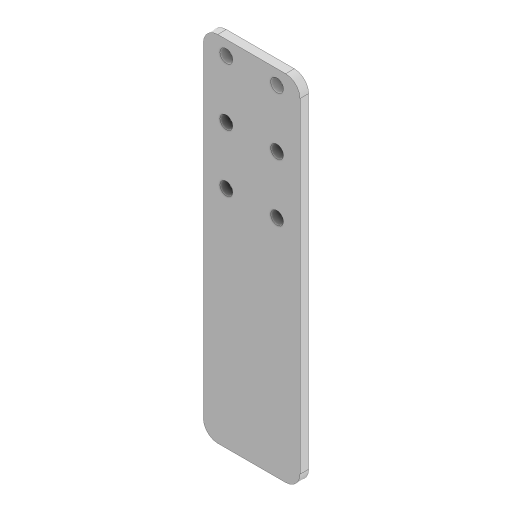
# Autodesk Inventor part: Lower Leaf
Saved by Autodesk Inventor 2024 (Build 280153000, 153)
## iProperties
Created: 2025-04-26
Part Number: Lower Leaf
Material: Generic
Document SubType Name: Modeling
Designer: Binara
Density: 1 g/cm^3
Appearance: Default
Author: Binara
Autodesk Inventor part; units mm, degrees
ref_plane "YZ Plane" through (0, 0, 0) normal (1, 0, 0) x (0, 1, 0)
ref_plane "XZ Plane" through (0, 0, 0) normal (0, 1, 0) x (-1, 0, 0)
ref_plane "XY Plane" through (0, 0, 0) normal (0, 0, 1) x (1, 0, 0)
sketch "Block1" plane through (0, 0, 0) normal (0, 0, 1) x (1, 0, 0)
  line L0 (22.2625, 0.2735) -> (22.2625, -13.7265)
  line L1 (56.7335, -13.7265) -> (22.2625, -13.7265)
  circle A0 centre (36.0618, -8.7265) radius 2.25
  circle A1 centre (53.7335, -8.7265) radius 2.25
  line L2 (61.7335, 0.2735) -> (61.7335, -8.7265)
  arc A2 (56.7335, -13.7265) -> (61.7335, -8.7265) centre (56.7335, -8.7265) ccw
  circle A3 centre (53.7335, 11.2735) radius 2.25
  line L3 (61.7335, 20.2735) -> (61.7335, 2.2735)
  circle A4 centre (36.0618, 11.2735) radius 2.25
  line L4 (61.7335, 0.2735) -> (22.2625, 0.2735)
  line L5 (22.2625, 2.2735) -> (61.7335, 2.2735)
  line L6 (22.2625, 20.2735) -> (22.2625, 2.2735)
  line L7 (61.7335, 31.2735) -> (61.7335, 22.2735)
  line L8 (61.7335, 20.2735) -> (22.2625, 20.2735)
  line L9 (22.2625, 22.2735) -> (61.7335, 22.2735)
  circle A5 centre (36.0618, 31.2735) radius 2.25
  line L10 (56.7335, 36.2735) -> (22.2625, 36.2735)
  line L11 (22.2625, 36.2735) -> (22.2625, 22.2735)
  circle A6 centre (53.7335, 31.2735) radius 2.25
  arc A7 (61.7335, 31.2735) -> (56.7335, 36.2735) centre (56.7335, 31.2735) ccw
  point P0 (44.3211, 11.7121)
  point P1 (21.7335, 36.2735)
sketch "Sketch1" plane through (0, 0, 0) normal (0, 0, 1) x (1, 0, 0)
  line L0 (57.9999, 40.92) -> (18.5289, 40.92)
  line L1 (18.5289, 40.92) -> (18.5289, -77.4287)
  line L2 (18.5289, -77.4287) -> (57.9999, -77.4287)
  line L3 (57.9999, -77.4287) -> (57.9999, 40.92)
  line L4 (24.3282, 45.92) -> (24.3282, -77.4287)
  line L5 (18.5289, 9.92) -> (18.5289, -4.08)
  line L6 (52.9999, -4.08) -> (18.5289, -4.08)
  circle A0 centre (32.3282, 0.92) radius 2.25
  circle A1 centre (49.9999, 0.92) radius 2.25
  line L7 (57.9999, 9.92) -> (57.9999, 0.92)
  arc A2 (52.9999, -4.08) -> (57.9999, 0.92) centre (52.9999, 0.92) ccw
  circle A3 centre (49.9999, 20.92) radius 2.25
  line L8 (57.9999, 29.92) -> (57.9999, 11.92)
  circle A4 centre (32.3282, 20.92) radius 2.25
  line L9 (57.9999, 9.92) -> (18.5289, 9.92)
  line L10 (18.5289, 11.92) -> (57.9999, 11.92)
  line L11 (18.5289, 29.92) -> (18.5289, 11.92)
  line L12 (57.9999, 40.92) -> (57.9999, 31.92)
  line L13 (57.9999, 29.92) -> (18.5289, 29.92)
  line L14 (18.5289, 31.92) -> (57.9999, 31.92)
  circle A5 centre (32.3282, 40.92) radius 2.25
  line L15 (52.9999, 45.92) -> (18.5289, 45.92)
  line L16 (18.5289, 45.92) -> (18.5289, 31.92)
  circle A6 centre (49.9999, 40.92) radius 2.25
  arc A7 (57.9999, 40.92) -> (52.9999, 45.92) centre (52.9999, 40.92) ccw
  point P0 (0, 0)
  point P1 (18.5289, 40.92)
  dimension "d3" = 8
  constraints: 10 end point, 2 parallel, 2 perpendicular, 1 horizontal, 1 point on line, 3 other
extrude "Extrusion1" add sketch "Sketch1" along normal blind 3 contours L3 L14 L4 L0 A5 A6 | L0 A6 A5 L4 L15 A7 | L3 L13 L4 L14 | L3 L10 L4 L13 | L3 L9 L4 L10 | L3 A2 L6 L4 L9 | L3 L2 L4 L6 A2
fillet "Fillet1" radius 5 3 edges at (57.9999, -77.4287, 1.5) (24.3282, -77.4287, 1.5) (24.3282, 45.92, 1.5)
body "Solid1"
